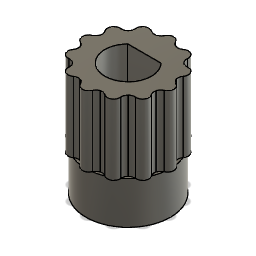
Shaft link (Autodesk Fusion 360 design; units mm, degrees)
Autodesk Fusion 360 part; units mm, degrees
note: some values were not read from the file. Set by a fixed rule: which sketch regions a step uses.
sketch "Sketch1" plane through (0, 0, 0) normal (0, 1, 0) x (1, 0, 0)
  circle A0 centre (0, 0) radius 3
  line L0 (0, -1.5) -> (0, 1)
  line L1 (0, 1) -> (1.118, 1)
  line L2 (1.118, 1) -> (-1.118, 1)
  arc A1 (-1.118, 1) -> (1.118, 1) centre (0, 0) ccw
  line L3 (1.1832, 1.15) -> (-1.1832, 1.15)
  arc A2 (-1.1832, 1.15) -> (1.1832, 1.15) centre (0, 0) ccw
  dimension "d1" = 3
  dimension "d2" = 6
  dimension "d3" = 2.5
  dimension "d4" = 1
  dimension "d5" = 0.15
  constraint coincident A0.centre A1.centre
  constraint concentric A0 A1
  constraint coincident L0.start A1
  constraint vertical L0
  constraint perpendicular L0 L1
  constraint perpendicular L0 L2
  measures "d1" diameter of A1
  measures "d2" diameter of A0
  measures "d3" distance of L0.start L0.end
  measures "d4" distance of A0.centre L2
extrude "Extrude1" add sketch "Sketch1" along normal blind 10 contours A0
sketch "Sketch2" plane through (0, 10, 0) normal (0, 1, 0) x (-1, 0, 0)
  arc A0 (1.1832, -1.15) -> (-1.1832, -1.15) centre (0, 0) ccw
  line L0 (1.1832, -1.15) -> (-1.1832, -1.15)
  circle A1 centre (0, 0) radius 3
  circle A2 centre (0, 0) radius 3.4
  arc A3 (1.1264, -2.7804) -> (1.846, -2.3647) centre (1.4009, -2.425) ccw
  arc A4 (-0.3896, -2.9697) -> (0.3896, -2.9697) centre (0, -2.8) ccw
  arc A5 (1.9745, -1.9852) -> (1.9852, -1.9745) centre (0, 0) ccw
  arc A6 (0.6911, -2.7134) -> (0.7335, -2.7022) centre (0, 0) ccw
  arc A7 (1.1264, -2.7804) -> (0.7335, -2.7022) centre (0.8514, -3.1365) ccw
  arc A8 (0.6911, -2.7134) -> (0.3896, -2.9697) centre (0.8022, -3.1494) ccw
  arc A9 (-0.3896, -2.9697) -> (-0.6911, -2.7134) centre (-0.8022, -3.1494) ccw
  arc A10 (1.9745, -1.9852) -> (1.846, -2.3647) centre (2.2919, -2.3043) ccw
  arc A11 (2.3646, -1.8459) -> (2.7809, -1.1248) centre (2.4249, -1.4) ccw
  arc A12 (2.9708, -0.4163) -> (2.9708, 0.4163) centre (2.8, 0) ccw
  arc A13 (2.7809, 1.1248) -> (2.3646, 1.8459) centre (2.4249, 1.4) ccw
  arc A14 (1.8459, 2.3646) -> (1.1248, 2.7809) centre (1.4, 2.4249) ccw
  arc A15 (0.4163, 2.9708) -> (-0.4485, 2.7638) centre (0, 2.8) ccw
  arc A16 (2.3646, -1.8459) -> (1.9852, -1.9745) centre (2.3043, -2.2919) ccw
  arc A17 (2.7065, 0.7174) -> (2.7026, 0.732) centre (0, 0) ccw
  arc A18 (2.7026, -0.732) -> (2.7065, -0.7174) centre (0, 0) ccw
  arc A19 (2.9708, -0.4163) -> (2.7065, -0.7174) centre (3.1415, -0.8327) ccw
  arc A20 (2.7026, -0.732) -> (2.7809, -1.1248) centre (3.137, -0.8496) ccw
  arc A21 (2.7065, 0.7174) -> (2.9708, 0.4163) centre (3.1415, 0.8327) ccw
  arc A22 (2.7809, 1.1248) -> (2.7026, 0.732) centre (3.137, 0.8496) ccw
  arc A23 (1.9852, 1.9745) -> (1.9745, 1.9852) centre (0, 0) ccw
  arc A24 (0.7335, -2.7022) -> (1.9745, -1.9852) centre (0, 0) ccw
  arc A25 (1.9852, 1.9745) -> (2.3646, 1.8459) centre (2.3043, 2.2919) ccw
  arc A26 (1.8459, 2.3646) -> (1.9745, 1.9852) centre (2.2919, 2.3043) ccw
  arc A27 (0.732, 2.7026) -> (0.7174, 2.7065) centre (0, 0) ccw
  arc A28 (0.732, 2.7026) -> (1.1248, 2.7809) centre (0.8496, 3.137) ccw
  arc A29 (0.4163, 2.9708) -> (0.7174, 2.7065) centre (0.8327, 3.1415) ccw
  line L1 (0, -4) -> (0, 4.5)
  arc A30 (-0.3896, -2.9697) -> (0.3896, -2.9697) centre (0, -2.8) ccw
  arc A31 (-0.3896, -2.9697) -> (-0.6911, -2.7134) centre (-0.8022, -3.1494) ccw
  arc A32 (-1.9745, -1.9852) -> (-0.7335, -2.7022) centre (0, 0) ccw
  arc A33 (-0.7335, -2.7022) -> (-1.1264, -2.7804) centre (-0.8514, -3.1365) ccw
  arc A34 (-1.846, -2.3647) -> (-1.1264, -2.7804) centre (-1.4009, -2.425) ccw
  arc A35 (-1.846, -2.3647) -> (-1.9745, -1.9852) centre (-2.2919, -2.3043) ccw
  arc A36 (-1.9852, -1.9745) -> (-2.3646, -1.8459) centre (-2.3043, -2.2919) ccw
  arc A37 (-2.7809, -1.1248) -> (-2.3646, -1.8459) centre (-2.4249, -1.4) ccw
  arc A38 (-2.7809, -1.1248) -> (-2.7026, -0.732) centre (-3.137, -0.8496) ccw
  arc A39 (-2.7065, -0.7174) -> (-2.9708, -0.4163) centre (-3.1415, -0.8327) ccw
  arc A40 (-2.9708, 0.4163) -> (-2.9708, -0.4163) centre (-2.8, 0) ccw
  arc A41 (-2.9708, 0.4163) -> (-2.7065, 0.7174) centre (-3.1415, 0.8327) ccw
  arc A42 (-2.7026, 0.732) -> (-2.7809, 1.1248) centre (-3.137, 0.8496) ccw
  arc A43 (-2.3646, 1.8459) -> (-2.7809, 1.1248) centre (-2.4249, 1.4) ccw
  arc A44 (-1.1248, 2.7809) -> (-1.8459, 2.3646) centre (-1.4, 2.4249) ccw
  arc A45 (0.4485, 2.7638) -> (-0.4163, 2.9708) centre (0, 2.8) ccw
  circle A46 centre (0, 0) radius 3
  arc A47 (-2.3646, 1.8459) -> (-1.9852, 1.9745) centre (-2.3043, 2.2919) ccw
  arc A48 (-1.9745, 1.9852) -> (-1.8459, 2.3646) centre (-2.2919, 2.3043) ccw
  arc A49 (-1.1248, 2.7809) -> (-0.732, 2.7026) centre (-0.8496, 3.137) ccw
  arc A50 (-0.7174, 2.7065) -> (-0.4163, 2.9708) centre (-0.8327, 3.1415) ccw
  line L2 (-1.9745, 1.9852) -> (-1.9852, 1.9745)
  line L3 (-0.7174, 2.7065) -> (-0.732, 2.7026)
  line L4 (-2.7026, 0.732) -> (-2.7065, 0.7174)
  line L5 (-2.7065, -0.7174) -> (-2.7026, -0.732)
  line L6 (-1.9852, -1.9745) -> (-1.9745, -1.9852)
  line L7 (-0.6911, -2.7134) -> (-0.7335, -2.7022)
  dimension "d8" = 6.8
  dimension "d9" = 5.6
  dimension "d10" = 0.85
  dimension "d13" = 0.45
  dimension "d14" = 0.45
  dimension "d15" = 0.45
  dimension "d16" = 0.45
  dimension "d17" = 0.45
  dimension "d18" = 0.45
  dimension "d19" = 0.45
  dimension "d20" = 0.45
  dimension "d21" = 0.45
  dimension "d22" = 0.45
  dimension "d23" = 0.45
  dimension "d24" = 0.45
  dimension "d25" = 0.45
  constraint concentric A0 A2
  constraint concentric A0 A5
  constraint coincident A4.centre A5
  constraint concentric A5 A6
  constraint tangent A3 A7
  constraint tangent A6 A7
  constraint tangent A4 A8
  constraint tangent A6 A8
  constraint tangent A4 A9
  constraint tangent A5 A9
  constraint tangent A3 A10
  constraint tangent A5 A10
  constraint coincident A5 A15.end
  constraint coincident A5 A9.end
  constraint tangent A11 A16
  constraint tangent A5 A16
  constraint concentric A2 A17
  constraint concentric A17 A18
  constraint tangent A12 A19
  constraint tangent A18 A19
  constraint tangent A11 A20
  constraint tangent A18 A20
  constraint tangent A12 A21
  constraint tangent A17 A21
  constraint tangent A13 A22
  constraint tangent A17 A22
  constraint concentric A17 A23
  constraint concentric A23 A24
  constraint tangent A13 A25
  constraint tangent A23 A25
  constraint coincident A6.end A23
  constraint tangent A14 A26
  constraint tangent A23 A26
  constraint concentric A2 A27
  constraint coincident A12.centre A27
  constraint tangent A14 A28
  constraint tangent A27 A28
  constraint tangent A15 A29
  constraint tangent A27 A29
  constraint vertical L1
  constraint symmetric A1 L1 A46
  constraint symmetric A3 L1 A34
  constraint symmetric A4 L1 A30
  constraint symmetric A3.start L1 A33.end
  constraint symmetric A6.end L1 A32.end
  constraint symmetric A7 L1 A33
  constraint symmetric A4.end L1 A4.start
  constraint symmetric A6.start L1 A9.end
  constraint symmetric A8 L1 A31
  constraint symmetric A4.start L1 A4.end
  constraint symmetric A3.end L1 A34.start
  constraint symmetric A5.start L1 A32.start
  constraint symmetric A10 L1 A35
  constraint symmetric A11 L1 A37
  constraint symmetric A12 L1 A40
  constraint symmetric A13 L1 A43
  constraint symmetric A14 L1 A44
  constraint symmetric A15.end L1 A45.start
  constraint symmetric A15 L1 A45
  constraint symmetric A11.start L1 A36.end
  constraint symmetric A5.end L1 A36.start
  constraint symmetric A16 L1 A36
  constraint symmetric A12.start L1 A39.end
  constraint symmetric A18.end L1 A39.start
  constraint symmetric A19 L1 A39
  constraint symmetric A11.end L1 A37.start
  constraint symmetric A18.start L1 A38.end
  constraint symmetric A20 L1 A38
  constraint symmetric A12.end L1 A40.start
  constraint symmetric A17.start L1 A41.end
  constraint symmetric A21 L1 A41
  constraint symmetric A13.start L1 A42.end
  constraint symmetric A17.end L1 A42.start
  constraint symmetric A22 L1 A42
  constraint symmetric A24 L1 A32
  constraint symmetric A13.end L1 A43.start
  constraint symmetric A23.start L1 A47.end
  constraint symmetric A25 L1 A47
  constraint symmetric A14.start L1 A44.end
  constraint symmetric A23.end L1 A48.start
  constraint symmetric A26 L1 A48
  constraint symmetric A14.end L1 A44.start
  constraint symmetric A27.start L1 A49.end
  constraint symmetric A28 L1 A49
  constraint symmetric A15.start L1 A45.end
  constraint symmetric A27.end L1 A50.start
  constraint symmetric A29 L1 A50
  measures "d8" diameter of A2
  measures "d9" diameter of A5
  measures "d10" diameter of A4
  measures "d13" radius of A7
  measures "d14" radius of A8
  measures "d15" radius of A9
  measures "d16" radius of A10
  measures "d17" radius of A16
  measures "d18" radius of A19
  measures "d19" radius of A20
  measures "d20" radius of A21
  measures "d21" radius of A22
  measures "d22" radius of A25
  measures "d23" radius of A26
  measures "d24" radius of A28
  measures "d25" radius of A29
extrude "Extrude2" add sketch "Sketch2" along normal blind 5 contours A0 L0 A1 A4 A5 A6 A8 A16 A17 A18 A19 A20 A21 A22 A23 A24 A25 A26 A27 A28 A29 L1 A30 A46 | A0 L0 A1 A4 A9 L1 A30 A31 A32 A36 A38 A39 A41 A42 A46 A47 A48 A49 A50 L2 L3 L4 L5 L6 L7 | A1 A15 L1 A45 A46 | A1 A15 L1 A45 A46 | A1 A4 L1 A30 A46 | A1 A4 L1 A30 A46 | A1 A14 A46 | A1 A44 A46 | A1 A34 A46 | A1 A32 A33 A35 A46 | A1 A7 A10 A24 A46 | A1 A3 A46 | A1 A13 A46 | A1 A43 A46 | A1 A37 A46 | A1 A11 A46 | A1 A12 A46 | A1 A40 A46
extrude "Extrude3" cut 1 faces at (0.0747, 0, -1.7639) along direction (0, 1, 0) blind 7
